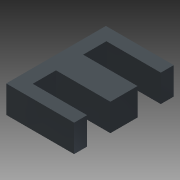
# Autodesk Inventor part: TSC_EL375
Saved by Autodesk Inventor 2015 (Build 190159000, 159)
## iProperties
Created: 2014-10-06
Part Number: TSC_EL375
Material: Iron, Gray
Document SubType Name: Modeling
Designer: Adam
Density: 7.15 g/cm^3
Appearance: Iron Gray
Author: Adam
Autodesk Inventor part; units mm, degrees
ref_plane "YZ Plane" through (0, 0, 0) normal (1, 0, 0) x (0, 1, 0)
sketch "Sketch1" plane through (0, 0, 0) normal (0, 1, 0) x (-1, 0, 0)
  line L0 (0, 0) -> (-4.75, 0)
  line L1 (-4.75, 0) -> (-4.75, -34.93)
  line L2 (-4.75, -34.93) -> (0, -34.93)
  line L3 (0, -34.93) -> (0, 0)
  line L4 (-4.75, 0) -> (-23.8, 0)
  line L5 (-23.8, 0) -> (-23.8, -4.565)
  line L6 (-23.8, -4.565) -> (-4.75, -4.565)
  line L7 (-4.75, -4.565) -> (-4.75, 0)
  line L8 (-4.75, -12.7) -> (-23.8, -12.7)
  line L9 (-23.8, -12.7) -> (-23.8, -22.23)
  line L10 (-23.8, -22.23) -> (-4.75, -22.23)
  line L11 (-4.75, -22.23) -> (-4.75, -12.7)
  line L12 (-4.75, -34.93) -> (-23.8, -34.93)
  line L13 (-23.8, -34.93) -> (-23.8, -30.365)
  line L14 (-23.8, -30.365) -> (-4.75, -30.365)
  line L15 (-4.75, -30.365) -> (-4.75, -34.93)
  line L16 (0, -17.465) -> (-23.9272, -17.465) construction
  point P0 (-23.8, -17.465)
  dimension "d0" = 34.93
  dimension "d1" = 9.53
  dimension "d2" = 25.8
  dimension "d3" = 12.9
  dimension "d4" = 19.05
  dimension "d5" = 23.8
  constraints: 34 end point, 8 parallel, 5 horizontal, 4 perpendicular, 4 point on line, 2 midpoint
  measures "d0" distance of L2.end L0.start
  measures "d1" distance of L8.end L9.end
  measures "d2" distance between parallel lines of L14 L6
  measures "d3" distance between parallel lines of L14 L16
  measures "d4" distance of L5.end L6.end
  measures "d5" distance between parallel lines of L3 L5
extrude "Extrusion1" add sketch "Sketch1" along normal blind 9.53
ref_plane "Work Plane2" through (0, 0, -17.465) normal (0, 0, 1) x (1, 0, 0)
ref_plane "Work Plane3" through (0, 4.765, 0) normal (0, -1, 0) x (1, 0, 0)
equation "\"d3\" = 0.5 * d2"
body "Solid1"
